Autodesk Inventor part; units mm, degrees
(part 2 of 2)
  spline S119 degree 2 poles (-59.5351, 70.2602) (-58.5197, 70.0389) (-57.6439, 69.5913) (-57.2445, 68.932) (-57.2445, 68.523) knots 0 0 0 1 2 3 3 3
  spline S120 degree 2 poles (-57.2445, 68.523) (-57.2445, 68.0417) (-57.7786, 67.2285) (-58.7315, 66.8098) (-59.4629, 66.8098) knots 0 0 0 1 2 3 3 3
  spline S121 degree 2 poles (-59.4629, 66.8098) (-60.7382, 66.8098) (-61.7247, 67.7915) (-61.7873, 68.5519) knots 0 0 0 1 2 2 2
  point P0 (0, 0)
  point P1 (-8, 83)
  point P2 (8, 83)
  point P3 (-83, 8)
  point P4 (83, 73)
  point P5 (83, 8)
  dimension "d46" = 45
  dimension "d47" = 20
  dimension "d48" = 40
  dimension "d49" = 20
  constraints: 2 horizontal alignment, 2 vertical, 2 vertical alignment, 1 midpoint, 4 other
  measures "d46" distance of L4.start L4.end
  measures "d47" distance of L6.end L4.start
  measures "d48" distance of L0.start L0.end
  measures "d49" distance of L0.end L1.end
extrude "Extrusion3" cut sketch "Sketch3" against normal blind 1
equation "\"d34\" = d33"
body "Solid1"
